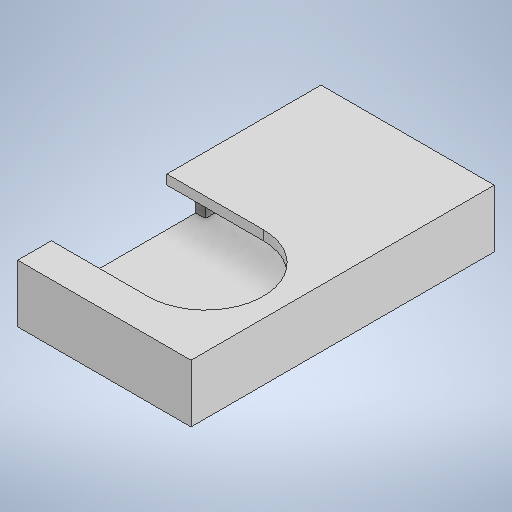
# Autodesk Inventor part: prototype2_2
Saved by Autodesk Inventor 2025.1 (Build 291241020, 241B)
## iProperties
Created: 2024-11-22
Part Number: prototype2_2
Material: Generic
Document SubType Name: Modeling
Designer: leon-
Density: 1 g/cm^3
Appearance: Default
Author: leon-
Autodesk Inventor part; units mm, degrees
ref_plane "YZ Plane" through (0, 0, 0) normal (1, 0, 0) x (0, 1, 0)
ref_plane "XZ Plane" through (0, 0, 0) normal (0, 1, 0) x (-1, 0, 0)
ref_plane "XY Plane" through (0, 0, 0) normal (0, 0, 1) x (1, 0, 0)
sketch "Sketch1" plane through (0, 0, 0) normal (0, 0, 1) x (1, 0, 0)
  line L0 (0, 0) -> (32, 0)
  line L1 (32, 0) -> (32, 8)
  line L2 (32, 8) -> (0, 8)
  line L3 (0, 8) -> (0, 0)
  line L4 (-2, 10) -> (34, 10)
  line L5 (34, 10) -> (34, -2)
  line L6 (34, -2) -> (-2, -2)
  line L7 (-2, -2) -> (-2, 10)
  dimension "d0" = 32
  dimension "d1" = 8
  dimension "d2" = 2
  dimension "d3" = 2
  dimension "d4" = 2
  dimension "d5" = 2
  constraints: 16 end point, 4 parallel, 2 horizontal, 2 perpendicular
  measures "d0" distance between parallel lines of L1 L3
  measures "d1" distance between parallel lines of L0 L2
  measures "d2" distance between parallel lines of L2 L4
  measures "d3" distance between parallel lines of L0 L6
  measures "d4" distance between parallel lines of L7 L3
  measures "d5" distance between parallel lines of L5 L1
extrude "Extrusion1" add sketch "Sketch1" along normal blind 60
sketch "Sketch3" plane through (0, 0, 60) normal (0, 0, 1) x (1, 0, 0)
  line L0 (34, 10) -> (-2, 10) projected
  line L1 (-2, -2) -> (34, -2) projected
  line L2 (34, -2) -> (34, 10) projected
  line L3 (34, 10) -> (-2, 10) projected
  line L4 (-2, 10) -> (-2, -2) projected
  line L5 (0, 0) -> (0, 8) projected
  line L6 (0, 8) -> (32, 8) projected
  line L7 (32, 8) -> (32, 0) projected
  line L8 (32, 0) -> (0, 0) projected
  point P0 (-2, 10)
extrude "Extrusion2" add sketch "Sketch3" along normal blind 3 contours L2 L1 L4 L0 | L5 L6 L7 L8
sketch "Sketch4" plane through (-2, -2, 0) normal (-1, 0, 0) x (0, 0, 1)
  line L0 (26, 2) -> (60, 2)
  line L1 (60, 2) -> (60, 10)
  line L2 (60, 10) -> (26, 10)
  line L3 (26, 10) -> (26, 2)
  line L4 (0, 12) -> (63, 12) projected
  line L5 (63, 12) -> (63, 0) projected
  point P0 (0, 2)
  point P1 (43, 10)
  dimension "d11" = 8
  dimension "d12" = 2
  dimension "d13" = 34
  dimension "d16" = 3
  constraints: 8 end point, 1 horizontal, 1 midpoint, 1 parallel
  measures "d11" distance from line of point (43, 10) L0
  measures "d12" distance between parallel lines of L4 L2
  measures "d13" distance between parallel lines of L1 L3
  measures "d16" distance between parallel lines of L5 L1
extrude "Extrusion3" cut sketch "Sketch4" against normal blind 3
sketch "Sketch2" plane through (-2, 10, 0) normal (0, 1, 0) x (1, 0, 0)
  line L0 (20, -44) -> (-20, -44) construction
  line L1 (20, -56) -> (-20, -56)
  line L2 (-20, -32) -> (20, -32)
  arc A0 (20, -56) -> (20, -32) centre (20, -44) ccw
  arc A1 (-20, -32) -> (-20, -56) centre (-20, -44) ccw
  line L3 (0, 0) -> (0, -63) projected
  point P0 (2, 0)
  point P1 (0, -44)
  point P2 (0, -26)
  point P3 (0, -60)
  point P4 (0, -32)
  point P5 (0, -56)
  dimension "d8" = 24
  dimension "d17" = 18
  dimension "d18" = 20
  dimension "d19" = 40
  constraints: 8 end point, 4 point on circle, 4 tangent, 2 centre point, 1 horizontal, 1 midpoint, 1 parallel
  measures "d8" distance between parallel lines of L1 L2
  measures "d17" distance from line of point (0, -26) L0
  measures "d18" distance from line of L3 L0.start
  measures "d19" distance of L2.start L2.end
extrude "Extrusion4" cut sketch "Sketch2" against normal blind 3 contours L1 L3 L2 A0
body "Solid1"
